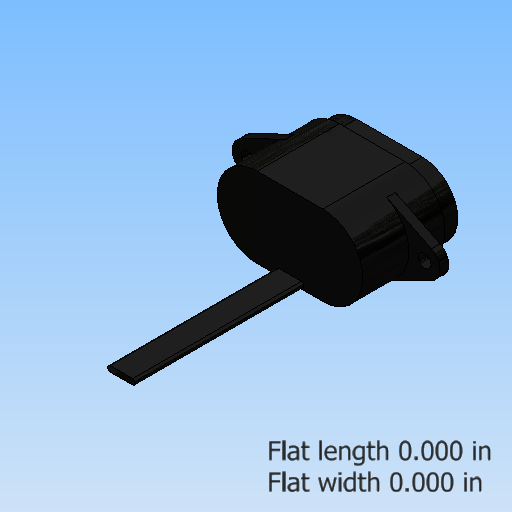
# Autodesk Inventor part: Cage Sensor
Saved by Autodesk Inventor 2025.4 (Build 294407000, 407)
## iProperties
RuleStatus: InUse
Created: 2025-10-10
Part Number: Cage Sensor
Material: Steel, Mild
Document SubType Name: Modeling
Designer: josh
Mass: 790.626 g
Surface Area: 2648.86 cm^2
Volume: 295.01 cm^3
Density: 7.85 g/cm^3
Sheet Metal Rule: Mild Steel .188
Sheet Metal Width: 0.000 in
Sheet Metal Length: 0.000 in
Sheet Metal Area: 0.000 in^2
Appearance: Default
Description: PROXIMITY SENSOR
AfterDocOpen0: PartNumber
Flat pattern length: =<Sheet Metal Length>
Flat pattern width: =<Sheet Metal Width>
Thickness: 0.188 in
Qty: 1
Flat Length: 0.0
Flat Width: 0.0
Part Area: 0.0
Author: josh
Autodesk Inventor part; units mm, degrees
ref_plane "YZ Plane" through (0, 0, 0) normal (1, 0, 0) x (0, 1, 0)
ref_plane "XZ Plane" through (0, 0, 0) normal (0, 1, 0) x (-1, 0, 0)
ref_plane "XY Plane" through (0, 0, 0) normal (0, 0, 1) x (1, 0, 0)
sketch "Sketch12" plane through (0, 0, 0) normal (0, 0, 1) x (1, 0, 0)
  line L0 (-7.4168, 0) -> (7.4168, 0) construction
  line L1 (-7.4168, -9.0424) -> (7.4168, -9.0424)
  line L2 (7.4168, 9.0424) -> (-7.4168, 9.0424)
  arc A0 (-7.4168, 9.0424) -> (-7.4168, -9.0424) centre (-7.4168, 0) ccw
  arc A1 (7.4168, -9.0424) -> (7.4168, 9.0424) centre (7.4168, 0) ccw
  circle A2 centre (-20.0152, 0) radius 1.4605
  line L3 (0, 0) -> (0, -9.0424)
  circle A3 centre (-20.0152, 0) radius 3.4798
  line L4 (-21.5516, -3.1222) -> (-11.4093, -8.1133)
  line L5 (-21.5516, 3.1222) -> (-11.4093, 8.1133)
  circle A4 centre (20.0152, 0) radius 1.4605
  circle A5 centre (20.0152, 0) radius 3.4798
  line L6 (21.5516, -3.1222) -> (11.4093, -8.1133)
  line L7 (21.5516, 3.1222) -> (11.4093, 8.1133)
  point P0 (16.4592, 0)
  point P1 (-16.4592, 0)
  point P2 (11.4093, -8.1133)
  point P3 (11.4093, 8.1133)
  dimension "d107" = 32.9184
  dimension "d108" = 18.0848
  dimension "d109" = 40.0304
  dimension "d110" = 2.921
  dimension "d111" = 46.99
  constraints: 18 end point, 12 point on circle, 8 tangent, 6 centre point, 5 symmetric about line, 2 midpoint, 1 horizontal, 1 horizontal alignment, 1 parallel, 2 other
  measures "d107" distance of point (16.459, 0) point (-16.459, 0)
  measures "d108" distance between parallel lines of L1 L2
  measures "d109" diameter of A2.centre L3
  measures "d110" diameter of A2
extrude "Extrusion1" add sketch "Sketch12" along normal mid plane 1.9558
sketch "Sketch13" plane through (0, 0, 0.9779) normal (0, 0, 1) x (1, 0, 0)
  arc A0 (-7.4168, 9.0424) -> (-7.4168, -9.0424) centre (-7.4168, 0) ccw projected
  arc A1 (7.4168, -9.0424) -> (7.4168, 9.0424) centre (7.4168, 0) ccw projected
  line L0 (7.4168, 9.0424) -> (-7.4168, 9.0424) projected
  line L1 (-7.4168, -9.0424) -> (7.4168, -9.0424) projected
  point P0 (0, 0)
extrude "Extrusion2" add sketch "Sketch13" along normal blind 10.414
sketch "Sketch14" plane through (0, 0, -0.9779) normal (0, 0, -1) x (-1, 0, 0)
  line L0 (7.4168, -9.0424) -> (-7.4168, -9.0424) projected
  arc A0 (-7.4168, 9.0424) -> (-7.4168, -9.0424) centre (-7.4168, 0) ccw projected
  line L1 (-7.4168, 9.0424) -> (7.4168, 9.0424) projected
  arc A1 (7.4168, -9.0424) -> (7.4168, 9.0424) centre (7.4168, 0) ccw projected
  point P0 (0, 0)
extrude "Extrusion3" add sketch "Sketch14" along normal blind 10.0965
sketch "Sketch15" plane through (0, 0, -11.0744) normal (0, 0, -1) x (-1, 0, 0)
  line L0 (-7.4168, -9.0424) -> (7.4168, -9.0424) projected
  arc A0 (7.4168, -9.0424) -> (7.4168, 9.0424) centre (7.4168, 0) ccw projected
  line L1 (7.4168, 9.0424) -> (-7.4168, 9.0424) projected
  arc A1 (-7.4168, 9.0424) -> (-7.4168, -9.0424) centre (-7.4168, 0) ccw projected
  line L2 (7.4168, -8.0137) -> (-7.4168, -8.0137)
  arc A2 (-7.4168, 8.0137) -> (-7.4168, -8.0137) centre (-7.4168, 0) ccw
  line L3 (-7.4168, 8.0137) -> (7.4168, 8.0137)
  arc A3 (7.4168, -8.0137) -> (7.4168, 8.0137) centre (7.4168, 0) ccw
  point P0 (0, 0)
  dimension "d118" = 16.0274
  constraints: 4 end point, 4 point on circle, 2 centre point, 3 other
  measures "d118" distance between parallel lines of L2 L3
extrude "Extrusion4" cut sketch "Sketch15" against normal blind 3.8862
sketch "Sketch16" plane through (0, 0, -11.0744) normal (0, 0, -1) x (-1, 0, 0)
  arc A0 (7.4168, -8.0137) -> (7.4168, 8.0137) centre (7.4168, 0) ccw projected
  line L0 (7.4168, 8.0137) -> (-7.4168, 8.0137) projected
  arc A1 (-7.4168, 8.0137) -> (-7.4168, -8.0137) centre (-7.4168, 0) ccw projected
  line L1 (-7.4168, -8.0137) -> (7.4168, -8.0137) projected
  circle A2 centre (7.4168, 0) radius 4.7625
  circle A3 centre (-7.4168, 0) radius 4.7625
  point P0 (0, 0)
  dimension "d121" = 9.525
  constraints: 2 centre point, 2 coincident, 1 equal radius
  measures "d121" diameter of A3
extrude "Extrusion5" add sketch "Sketch16" along normal blind 0.254 contours A2 | A3
sketch "Sketch17" plane through (0, 0, 11.3919) normal (0, 0, 1) x (1, 0, 0)
  line L0 (-7.4168, -9.0424) -> (7.4168, -9.0424) projected
  line L1 (2.54, -8.1534) -> (-2.54, -8.1534) construction
  line L2 (2.54, -7.5184) -> (-2.54, -7.5184)
  line L3 (-2.54, -8.7884) -> (2.54, -8.7884)
  arc A0 (2.54, -8.7884) -> (2.54, -7.5184) centre (2.54, -8.1534) ccw
  arc A1 (-2.54, -7.5184) -> (-2.54, -8.7884) centre (-2.54, -8.1534) ccw
  point P0 (0, 0)
  point P1 (0, -8.1534)
  point P2 (0, -8.7884)
  point P3 (0, -9.0424)
  dimension "d124" = 5.08
  dimension "d125" = 0.254
  dimension "d126" = 1.27
  constraints: 8 end point, 4 point on circle, 4 tangent, 3 midpoint, 2 centre point, 2 parallel, 1 vertical alignment
  measures "d124" distance of L1.start L1.end
  measures "d125" distance between parallel lines of L3 L0
  measures "d126" distance between parallel lines of L2 L3
extrude "Extrusion6" add sketch "Sketch17" along normal blind 38.1
equation "\"BendRadius\" = Thickness"
equation "\"BendReliefWidth\" = Thickness"
equation "\"BendReliefDepth\" = 0.5 * Thickness"
equation "\"CornerReliefSize\" = 4 * Thickness"
equation "\"MinimumRemnant\" = 2 * Thickness"
equation "\"TransitionRadius\" = BendRadius"
equation "\"JacobiRadiusSize\" = BendRadius"
equation "\"GapSize\" = Thickness"
equation "\"Thickness\" = 4.7625"
body "Solid3"
